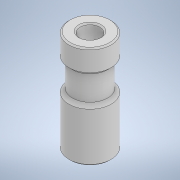
# Autodesk Inventor part: prostavka
Saved by Autodesk Inventor 2021 (Build 250183000, 183)
## iProperties
Created: 2023-02-07
Part Number: prostavka
Material: Типовые
Document SubType Name: Modeling
Designer: ignat
Density: 1 g/cm^3
Appearance: По умолчанию
Author: ignat
Autodesk Inventor part; units mm, degrees
ref_plane "YZ Plane" through (0, 0, 0) normal (1, 0, 0) x (0, 1, 0)
ref_plane "XZ Plane" through (0, 0, 0) normal (0, 1, 0) x (-1, 0, 0)
ref_plane "XY Plane" through (0, 0, 0) normal (0, 0, 1) x (1, 0, 0)
sketch "Эскиз1" plane through (0, 0, 0) normal (1, 0, 0) x (0, 1, 0)
  line L0 (0, 2.8) -> (29, 2.8)
  line L1 (0, 6) -> (15, 6)
  line L2 (15, 6) -> (15, 5)
  line L3 (22, 5) -> (22, 6)
  line L4 (22, 6) -> (29, 6)
  line L5 (29, 6) -> (29, 2.8)
  line L6 (22, 5) -> (15, 5)
  line L7 (0, 6) -> (0, 2.8)
  line L8 (32.1482, 0) -> (-3.0834, 0)
  point P0 (0, 0)
  constraints: 18 end point, 3 perpendicular, 2 horizontal, 2 vertical
revolve "Вращение1" add sketch "Эскиз1" angle 360 about axis through (0, 32.1482, 0) along (0, -1, 0)
chamfer "Фаска1" distance 1 angle 45 2 edges at (0, 15, -6) (0, 22, -6)
chamfer "Фаска2" distance 0.4 angle 45 4 edges at (0, 29, -2.8) (0, 29, -6) (0, 0, -6) (0, 0, -2.8)
